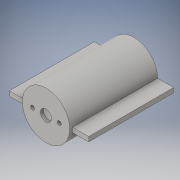
# Autodesk Inventor part: Attachment2
Saved by Autodesk Inventor 2016 SP1 (Build 200210100, 210)
## iProperties
Created: 2016-04-13
Part Number: Attachment2
Material: Generic
Document SubType Name: Modeling
Designer: schiu30
Density: 1 g/cm^3
Appearance: Default
Author: schiu30
Autodesk Inventor part; units mm, degrees
ref_plane "YZ Plane" through (0, 0, 0) normal (1, 0, 0) x (0, 1, 0)
ref_plane "XZ Plane" through (0, 0, 0) normal (0, 1, 0) x (-1, 0, 0)
ref_plane "XY Plane" through (0, 0, 0) normal (0, 0, 1) x (1, 0, 0)
sketch "Sketch1" plane through (0, 0, 0) normal (0, 0, 1) x (1, 0, 0)
  line L0 (-25.1968, 0) -> (-25.1968, -2.9718)
  line L1 (-25.1968, -2.9718) -> (-14.7402, -2.9718)
  line L2 (25.1968, 0) -> (25.1968, -2.9718)
  line L3 (25.1968, -2.9718) -> (14.7402, -2.9718)
  line L4 (-25.1968, 0) -> (-15.0368, 0)
  line L5 (15.0368, 0) -> (25.1968, 0)
  circle A0 centre (0, 0) radius 12.4968
  arc A1 (15.0368, 0) -> (-15.0368, 0) centre (0, 0) ccw
  arc A2 (-14.7402, -2.9718) -> (14.7402, -2.9718) centre (0, 0) ccw
  point P0 (-12.4968, 0)
  dimension "d12" = 24.9936
  dimension "d4" = 2.9718
  dimension "d5" = 2.9718
  dimension "d6" = 50.3936
  dimension "d9" = 12.7
  dimension "d13" = 15.0368
  dimension "d14" = 15.0368
  dimension "d15" = 10.4566
  dimension "d16" = 10.4566
  dimension "d17" = 10.16
  constraints: 12 end point, 4 point on circle, 2 centre point, 2 coincident, 2 horizontal, 2 point on line, 1 horizontal alignment, 1 perpendicular, 1 vertical, 2 other
  measures "d4" distance of L0.start L0.end
  measures "d5" distance of L2.start L2.end
  measures "d6" distance of L0.start L2.start
  measures "d9" distance of L0.start point (-12.497, 0)
  measures "d13" radius of A1
  measures "d14" radius of A2
  measures "d15" distance of L0.end L1.end
  measures "d16" distance of L2.end L3.end
  measures "d17" distance of L5.start L2.start
extrude "Extrusion2" add sketch "Sketch1" along normal blind 53.975
sketch "Sketch2" plane through (0, 0, 53.975) normal (0, 0, 1) x (1, 0, 0)
  circle A0 centre (0, 0) radius 3.556
  circle A1 centre (0, 0) radius 15.0368
  dimension "d20" = 7.112
  dimension "d21" = 30.0736
  constraints: 2 centre point, 1 coincident
  measures "d20" diameter of A0
  measures "d21" diameter of A1
extrude "Extrusion3" add sketch "Sketch2" along normal blind 1.905
sketch "Sketch3" plane through (0, 0, 55.88) normal (0, 0, 1) x (1, 0, 0)
  circle A0 centre (0, 0) radius 12.4968 projected
  circle A1 centre (-8.4968, 0) radius 1.25
  circle A2 centre (8.4968, 0) radius 1.25
  dimension "d25" = 2.5
  dimension "d26" = 8.4968
  dimension "d27" = 2.5
  dimension "d28" = 8.4968
  constraints: 2 centre point
  measures "d25" diameter of A1
  measures "d26" distance of A1.centre A0.centre
  measures "d27" diameter of A2
  measures "d28" distance of A0.centre A2.centre
extrude "Extrusion4" cut sketch "Sketch3" against normal blind 254 contours A1 | A2
body "Solid2"
